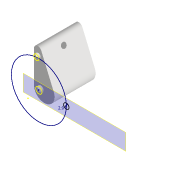
# Autodesk Inventor part: Anglerfish_coverslipclamp_levelarm
Saved by Autodesk Inventor 2022 (Build 260153000, 153)
## iProperties
Created: 2023-04-11
Part Number: Anglerfish_coverslipclamp_levelarm
Material: Generisch
Document SubType Name: Modeling
Designer: diederichbenedict
Density: 1 g/cm^3
Appearance: Vorgabe
Author: diederichbenedict
Autodesk Inventor part; units mm, degrees
ref_plane "YZ Plane" through (0, 0, 0) normal (1, 0, 0) x (0, 1, 0)
ref_plane "XZ Plane" through (0, 0, 0) normal (0, 1, 0) x (-1, 0, 0)
ref_plane "XY Plane" through (0, 0, 0) normal (0, 0, 1) x (1, 0, 0)
sketch "Skizze1" plane through (0, 0, 0) normal (0, 0, 1) x (1, 0, 0)
  circle A0 centre (5.8119, 6.7241) radius 1.5 projected
  circle A1 centre (7.8119, 6.7241) radius 5.5
  line L0 (2.3119, 6.7241) -> (2.3119, 24.7241)
  line L1 (4.3119, 26.7241) -> (5.3119, 26.7241)
  line L2 (5.3119, 26.7241) -> (12.8762, 8.8696)
  arc A2 (4.3119, 26.7241) -> (2.3119, 24.7241) centre (4.3119, 24.7241) ccw
  circle A3 centre (5.8119, 6.7241) radius 1.7
  point P0 (0, 0)
  point P1 (2.3119, 26.7241)
  dimension "d0" = 20
  dimension "d1" = 3
  dimension "d2" = 2
  dimension "d3" = 2
  dimension "d6" = 0.2
  dimension "d14" = 11
  constraints: 6 end point, 4 point on circle, 4 tangent, 3 centre point, 2 point on line, 1 perpendicular, 1 vertical
  measures "d0" distance of L0.start point (2.312, 26.724)
  measures "d1" distance of point (2.312, 26.724) L1.end
  measures "d2" distance of A1.centre A0.centre
  measures "d3" radius of A2
  measures "d6" radial gap between concentric circles of A0 A3
  measures "d14" diameter of A1
extrude "Extrusion1" add sketch "Skizze1" along normal blind 22 contours A1 | A1 L0 A2 L1 L2
fillet "Rundung1" radius 2 1 edges at (5.3119, 26.7241, 11)
sketch "Skizze2" plane through (0, 0, 0) normal (0, 0, -1) x (-1, 0, 0)
  circle A0 centre (-5.8119, 6.7241) radius 1.7 projected
  arc A1 (-2.3119, 23.9575) -> (-6.1535, 24.7377) centre (-4.3119, 23.9575) ccw projected
  line L0 (-12.8762, 8.8696) -> (-6.1535, 24.7377) projected
  arc A2 (-12.8762, 8.8696) -> (-2.3119, 6.7241) centre (-7.8119, 6.7241) ccw projected
  line L1 (-2.3119, 23.9575) -> (-2.3119, 6.7241) projected
  circle A3 centre (-4.5041, 21.3778) radius 1.45
  point P0 (0, 0)
  dimension "d8" = 2.9
  constraints: 1 centre point
  measures "d8" diameter of A3
extrude "Extrusion2" cut sketch "Skizze2" against normal blind 4 contours A3
sketch "Skizze3" plane through (0, 0, 22) normal (0, 0, 1) x (1, 0, 0)
  circle A0 centre (4.5041, 21.3778) radius 1.45 projected
  point P0 (0, 0)
extrude "Extrusion3" cut sketch "Skizze3" against normal blind 4
ref_plane "Arbeitsebene1" through (50, 0, 23) normal (0, 0, -1) x (-1, 0, 0)
sketch "Skizze4" plane through (50, 0, 23) normal (0, 0, -1) x (-1, 0, 0)
  circle A0 centre (45.4959, 21.3778) radius 1.45 projected
  circle A1 centre (44.1881, 6.7241) radius 1.7 projected
  circle A2 centre (44.1881, 6.7241) radius 1.7 projected
  circle A3 centre (45.4959, 21.3778) radius 1.45 projected
  circle A4 centre (44.1881, 6.7241) radius 14.712
  circle A5 centre (29.4761, 6.7241) radius 1.45
  point P0 (50, 0)
  dimension "d13" = 2.9
  constraints: 2 centre point, 2 point on circle, 1 coincident
  measures "d13" diameter of A5
sketch "Skizze5" plane through (12.8762, 8.8696, 22) normal (0.9208, 0.3901, 0) x (0, 0, -1)
  line L0 (0, 17.2334) -> (22, 17.2334) projected
  line L1 (0, 0) -> (0, 17.2334) projected
  line L2 (22, 0) -> (0, 0) projected
  line L3 (22, 0) -> (22, 17.2334) projected
  circle A0 centre (11, 14.4172) radius 1.4
  point P0 (22, -3.1439)
  dimension "d15" = 2.8
  constraints: 1 centre point
  measures "d15" diameter of A0
extrude "Extrusion4" cut sketch "Skizze5" against normal blind 10 contours A0
